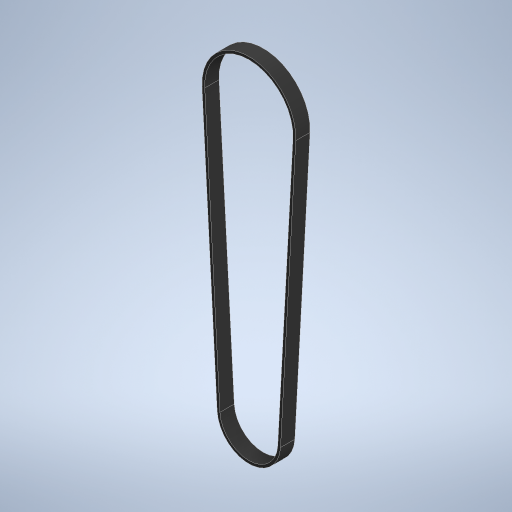
# Autodesk Inventor part: 9mm_belt
Saved by Autodesk Inventor 2024 (Build 280153000, 153)
## iProperties
Created: 2024-12-23
Part Number: 9mm_belt
Material: Rubber
Document SubType Name: Modeling
Designer: Danielle
Density: 0.93 g/cm^3
Appearance: Rubber - Black
Author: Danielle
Autodesk Inventor part; units mm, degrees
ref_plane "YZ Plane" through (0, 0, 0) normal (1, 0, 0) x (0, 1, 0)
ref_plane "XZ Plane" through (0, 0, 0) normal (0, 1, 0) x (-1, 0, 0)
ref_plane "XY Plane" through (0, 0, 0) normal (0, 0, 1) x (1, 0, 0)
sketch "Sketch1" plane through (0, 0, 0) normal (0, 0, 1) x (1, 0, 0)
  circle A0 centre (0, 0) radius 19.1008 construction
  circle A1 centre (0, 172.4406) radius 28.6512 construction
  line L0 (-28.6072, 170.8538) -> (-19.0715, -1.0579) construction
  line L1 (19.0715, -1.0579) -> (28.6072, 170.8538) construction
  arc A2 (28.6072, 170.8538) -> (-28.6072, 170.8538) centre (0, 172.4406) ccw construction
  arc A3 (-19.0715, -1.0579) -> (19.0715, -1.0579) centre (0, 0) ccw construction
  line L2 (29.4759, 170.8056) -> (19.9401, -1.1061)
  arc A4 (-19.9401, -1.1061) -> (19.9401, -1.1061) centre (0, 0) ccw
  line L3 (-19.9401, -1.1061) -> (-29.4759, 170.8056)
  arc A5 (29.4759, 170.8056) -> (-29.4759, 170.8056) centre (0, 172.4406) ccw
  line L4 (27.7386, 170.902) -> (18.2028, -1.0097)
  arc A6 (-18.2028, -1.0097) -> (18.2028, -1.0097) centre (0, 0) ccw
  line L5 (-18.2028, -1.0097) -> (-27.7386, 170.902)
  arc A7 (27.7386, 170.902) -> (-27.7386, 170.902) centre (0, 172.4406) ccw
  dimension "d0" = 172.4406
  dimension "d1" = 38.2016
  dimension "d2" = 57.3024
  dimension "d3" = 0.87
  dimension "d4" = 0.87
  constraints: 16 point on circle, 12 end point, 8 centre point, 7 tangent, 1 coincident, 1 vertical alignment, 6 other
  measures "d0" distance of point (0, 0) A1.centre
  measures "d1" diameter of A0
  measures "d2" diameter of A1
  measures "d3" distance between parallel lines of L1 L2
  measures "d4" distance between parallel lines of L1 L4
extrude "Extrusion1" add sketch "Sketch1" along normal blind 9
body "Solid1"
